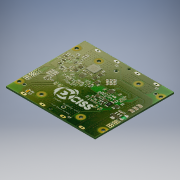
# Autodesk Inventor part: PSU-PCB
Saved by Autodesk Inventor 2017 (Build 210142000, 142)
## iProperties
Part Number: PSU-PCB
Material: Generisch
Document SubType Name: Modeling
Designer: David
Density: 1 g/cm^3
Appearance: Dunkelgrün
Author: David
Autodesk Inventor part; units mm, degrees
ref_plane "YZ Plane" through (0, 0, 0) normal (1, 0, 0) x (0, 1, 0)
ref_plane "XZ Plane" through (0, 0, 0) normal (0, 1, 0) x (-1, 0, 0)
ref_plane "XY Plane" through (0, 0, 0) normal (0, 0, 1) x (1, 0, 0)
sketch "Skizze1" plane through (0, 0, 0) normal (0, 0, 1) x (1, 0, 0)
  line L0 (0, 0) -> (90.4, 0)
  line L1 (90.4, 0) -> (90.4, 80)
  line L2 (90.4, 80) -> (0, 80)
  line L3 (0, 80) -> (0, 0)
  line L4 (2.6, 69.1) -> (87.8, 69.1) construction
  line L5 (87.8, 69.1) -> (87.8, 10.9) construction
  line L6 (87.8, 10.9) -> (2.6, 10.9) construction
  line L7 (2.6, 10.9) -> (2.6, 69.1) construction
  circle A0 centre (2.6, 69.1) radius 1.6
  circle A1 centre (2.6, 10.9) radius 1.6
  circle A2 centre (87.8, 69.1) radius 1.6
  circle A3 centre (87.8, 10.9) radius 1.6
  line L8 (25.2, 40) -> (65.2, 40) construction
  line L9 (65.2, 69.1) -> (65.2, 10.9) construction
  line L10 (65.2, 10.9) -> (47.65, 10.9) construction
  line L11 (65.2, 69.1) -> (82.75, 69.1) construction
  line L12 (25.2, 69.1) -> (25.2, 10.9) construction
  line L13 (25.2, 69.1) -> (42.75, 69.1) construction
  line L14 (25.2, 10.9) -> (7.65, 10.9) construction
  circle A4 centre (7.65, 10.9) radius 1.225
  circle A5 centre (42.75, 69.1) radius 1.225
  circle A6 centre (82.75, 69.1) radius 1.225
  circle A7 centre (47.65, 10.9) radius 1.225
  circle A8 centre (47.65, 77.32) radius 1.195
  circle A9 centre (42.75, 2.68) radius 1.195
  circle A10 centre (65.2, 10.9) radius 1.6
  circle A11 centre (65.2, 69.1) radius 1.6
  circle A12 centre (25.2, 69.1) radius 1.6
  circle A13 centre (25.2, 10.9) radius 1.6
  line L15 (1.9, 19.45) -> (3.9, 19.45) construction
  line L16 (3.9, 19.45) -> (3.9, 17.45) construction
  line L17 (3.9, 17.45) -> (1.9, 17.45) construction
  line L18 (1.9, 17.45) -> (1.9, 19.45) construction
  line L19 (1.9, 25.15) -> (3.9, 25.15) construction
  line L20 (3.9, 25.15) -> (3.9, 23.15) construction
  line L21 (3.9, 23.15) -> (1.9, 23.15) construction
  line L22 (1.9, 23.15) -> (1.9, 25.15) construction
  line L23 (1.8, 30.1) -> (4.2, 30.1) construction
  line L24 (4.2, 30.1) -> (4.2, 27.9) construction
  line L25 (4.2, 27.9) -> (1.8, 27.9) construction
  line L26 (1.8, 27.9) -> (1.8, 30.1) construction
  line L27 (2.9, 19.45) -> (2.9, 23.15) construction
  circle A14 centre (1.9, 23.15) radius 0.5588
  circle A15 centre (3.9, 23.15) radius 0.5588
  circle A16 centre (3.9, 25.15) radius 0.5588
  circle A17 centre (1.9, 25.15) radius 0.5588
  circle A18 centre (1.9, 19.45) radius 0.5588
  circle A19 centre (3.9, 19.45) radius 0.5588
  circle A20 centre (3.9, 17.45) radius 0.5588
  circle A21 centre (1.9, 17.45) radius 0.5588
  line L28 (1.8, 27.9) -> (4.2, 30.1) construction
  circle A22 centre (4.2, 27.9) radius 0.4064
  circle A23 centre (1.8, 27.9) radius 0.4064
  circle A24 centre (4.2, 30.1) radius 0.4064
  circle A25 centre (1.8, 30.1) radius 0.4064
  line L29 (86.3, 19.45) -> (88.3, 19.45) construction
  line L30 (88.3, 19.45) -> (88.3, 17.45) construction
  line L31 (88.3, 17.45) -> (86.3, 17.45) construction
  line L32 (86.3, 17.45) -> (86.3, 19.45) construction
  line L33 (86.3, 25.15) -> (88.3, 25.15) construction
  line L34 (88.3, 25.15) -> (88.3, 23.15) construction
  line L35 (88.3, 23.15) -> (86.3, 23.15) construction
  line L36 (86.3, 23.15) -> (86.3, 25.15) construction
  line L37 (87.3, 19.45) -> (87.3, 23.15) construction
  circle A26 centre (86.3, 23.15) radius 0.5588
  circle A27 centre (88.3, 23.15) radius 0.5588
  circle A28 centre (88.3, 25.15) radius 0.5588
  circle A29 centre (86.3, 25.15) radius 0.5588
  circle A30 centre (86.3, 19.45) radius 0.5588
  circle A31 centre (88.3, 19.45) radius 0.5588
  circle A32 centre (88.3, 17.45) radius 0.5588
  circle A33 centre (86.3, 17.45) radius 0.5588
  line L38 (55.65, 77.61) -> (74.75, 77.61) construction
  line L39 (74.75, 77.61) -> (74.75, 2.39) construction
  line L40 (74.75, 2.39) -> (55.65, 2.39) construction
  line L41 (55.65, 2.39) -> (55.65, 77.61) construction
  circle A34 centre (55.65, 2.39) radius 0.66
  circle A35 centre (74.75, 2.39) radius 0.66
  circle A36 centre (74.75, 77.61) radius 0.66
  circle A37 centre (55.65, 77.61) radius 0.66
  line L42 (15.65, 77.61) -> (34.75, 77.61) construction
  line L43 (34.75, 77.61) -> (34.75, 2.39) construction
  line L44 (34.75, 2.39) -> (15.65, 2.39) construction
  line L45 (15.65, 2.39) -> (15.65, 77.61) construction
  circle A38 centre (15.65, 2.39) radius 0.66
  circle A39 centre (34.75, 2.39) radius 0.66
  circle A40 centre (34.75, 77.61) radius 0.66
  circle A41 centre (15.65, 77.61) radius 0.66
  line L46 (55.65, 2.39) -> (74.75, 77.61) construction
  line L47 (15.65, 2.39) -> (34.75, 77.61) construction
  line L48 (23.2, 29.27) -> (23.2, 26.73) construction
  circle A42 centre (23.2, 26.73) radius 0.45
  circle A43 centre (23.2, 29.27) radius 0.45
  line L49 (27.2, 29.27) -> (27.2, 26.73) construction
  circle A44 centre (27.2, 26.73) radius 0.45
  circle A45 centre (27.2, 29.27) radius 0.45
  line L50 (23.2, 28) -> (27.2, 28) construction
  line L51 (63.2, 29.27) -> (63.2, 26.73) construction
  circle A46 centre (63.2, 26.73) radius 0.45
  circle A47 centre (63.2, 29.27) radius 0.45
  circle A48 centre (67.2, 29.27) radius 0.45
  line L52 (67.2, 29.27) -> (67.2, 26.73) construction
  circle A49 centre (67.2, 26.73) radius 0.45
  line L53 (63.2, 28) -> (67.2, 28) construction
  point P0 (2.9, 21.3)
  point P1 (3, 29)
  point P2 (87.3, 21.3)
  dimension "d0" = 90.4
  dimension "d1" = 80
  dimension "d2" = 2.6
  dimension "d3" = 10.9
  dimension "d4" = 69.1
  dimension "d5" = 87.8
  dimension "d6" = 3.2
  dimension "d7" = 40
  dimension "d8" = 25.2
  dimension "d9" = 65.2
  dimension "d10" = 2.45
  dimension "d11" = 2.39
  dimension "d12" = 17.55
  dimension "d13" = 17.55
  dimension "d14" = 37.32
  dimension "d15" = 37.32
  dimension "d16" = 3.2
  dimension "d17" = 29.1
  dimension "d18" = 17.55
  dimension "d21" = 1.85
  dimension "d22" = 2
  dimension "d23" = 1.1176
  dimension "d24" = 2.4
  dimension "d25" = 2.2
  dimension "d26" = 0.8128
  dimension "d27" = 1.85
  dimension "d28" = 2
  dimension "d29" = 1.1176
  dimension "d30" = 2.9
  dimension "d31" = 3
  dimension "d32" = 21.3
  dimension "d33" = 29
  dimension "d34" = 87.3
  dimension "d35" = 21.3
  dimension "d36" = 1.32
  dimension "d37" = 19.1
  dimension "d38" = 75.22
  dimension "d39" = 1.32
  dimension "d40" = 19.1
  dimension "d41" = 75.22
  dimension "d42" = 0.9
  dimension "d43" = 2.54
  dimension "d44" = 0.9
  dimension "d45" = 2.54
  dimension "d46" = 4
  dimension "d47" = 0.9
  dimension "d48" = 2.54
  dimension "d49" = 0.9
  dimension "d50" = 2.54
  dimension "d51" = 4
  dimension "d52" = 28
  dimension "d53" = 23.2
  dimension "d54" = 63.2
  constraints: 108 end point, 50 centre point, 50 coincident, 37 equal radius, 18 parallel, 15 midpoint, 14 horizontal, 13 perpendicular, 10 equal length, 6 vertical, 1 collinear
  measures "d0" distance of L0.start L0.end
  measures "d1" distance of L0.end L1.end
  measures "d2" distance between parallel lines of L3 L7
  measures "d3" distance between parallel lines of L0 L6
  measures "d4" distance between parallel lines of L0 L4
  measures "d5" distance from line of L0.start L5
  measures "d6" diameter of A0
  measures "d7" distance between parallel lines of L8 L0
  measures "d8" distance from line of L8.start L3
  measures "d9" distance from line of L3 L8.end
  measures "d10" diameter of A5
  measures "d11" diameter of A8
  measures "d12" distance from line of A8.centre L9
  measures "d13" distance from line of A9.centre L12
  measures "d14" vertical distance of L8.end A8.centre
  measures "d15" vertical distance of L8.start A9.centre
  measures "d16" diameter of A11
  measures "d17" distance from line of L8.end L10
  measures "d18" distance of L9.start L11.end
  measures "d21" distance from line of L21 point (2.9, 21.3)
  measures "d22" distance of L20.end L21.end
  measures "d23" diameter of A16
  measures "d24" distance of L24.end L25.end
  measures "d25" distance of L23.end L24.end
  measures "d26" diameter of A24
  measures "d27" distance from line of L35 point (87.3, 21.3)
  measures "d28" distance of L35.start L35.end
  measures "d29" diameter of A28
  measures "d30" distance from line of L3 point (2.9, 21.3)
  measures "d31" distance from line of point (3, 29) L3
  measures "d32" distance from line of point (2.9, 21.3) L0
  measures "d33" distance from line of point (3, 29) L0
  measures "d34" distance from line of point (87.3, 21.3) L3
  measures "d35" distance from line of point (87.3, 21.3) L0
  measures "d36" diameter of A36
  measures "d37" distance of L39.end L40.end
  measures "d38" distance of L38.end L39.end
  measures "d39" diameter of A40
  measures "d40" distance of L44.start L44.end
  measures "d41" distance of L42.end L44.start
  measures "d42" diameter of A43
  measures "d43" distance of L48.start L48.end
  measures "d44" diameter of A45
  measures "d45" distance of L49.start L49.end
  measures "d46" distance of L50.start L50.end
  measures "d47" diameter of A47
  measures "d48" distance of L51.start L51.end
  measures "d49" diameter of A48
  measures "d50" distance of L52.start L52.end
  measures "d51" distance of L53.start L53.end
  measures "d52" distance between parallel lines of L50 L0
  measures "d53" distance from line of L50.start L3
  measures "d54" distance between parallel lines of L3 L51
extrude "Extrusion1" add sketch "Skizze1" along normal mid plane 1.6
sketch "Skizze2" plane through (0, 0, 0.8) normal (0, 0, 1) x (1, 0, 0)
  line L0 (0, 79.9165) -> (90.4, 79.9165) construction
  line L1 (90.4, 79.9165) -> (90.4, 0.0835) construction
  line L2 (90.4, 0.0835) -> (0, 0.0835) construction
  line L3 (0, 0.0835) -> (0, 79.9165) construction
  point P0 (90.4, 40)
  point P1 (0, 40)
  constraints: 2 midpoint, 2 other
decal "Aufkleber1"
equation "\"d13\" = d12"
equation "\"d15\" = d14"
